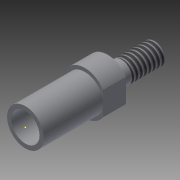
# Autodesk Inventor part: Fuel Adjuster
Saved by Autodesk Inventor 2015 (Build 190159000, 159)
## iProperties
Created: 2016-02-20
Part Number: Fuel Adjuster
Material: Generic
Document SubType Name: Modeling
Designer: Owner
Density: 1 g/cm^3
Appearance: Default
Author: Owner
Autodesk Inventor part; units mm, degrees
ref_plane "XZ Plane" through (0, 0, 0) normal (0, 1, 0) x (-1, 0, 0)
ref_plane "XY Plane" through (0, 0, 0) normal (0, 0, 1) x (1, 0, 0)
sketch "Sketch1" plane through (0, 0, 0) normal (0, 0, 1) x (1, 0, 0)
  circle A0 centre (0, 0) radius 1.9685
  dimension "d0" = 3.937
  constraints: 1 centre point, 1 coincident
  measures "d0" diameter of A0
extrude "Extrusion1" add sketch "Sketch1" along normal blind 8.636
sketch "Sketch2" plane through (0, 0, 8.636) normal (0, 0, 1) x (1, 0, 0)
  circle A0 centre (0, 0) radius 4.0005
  dimension "d3" = 8.001
  constraints: 1 centre point, 1 coincident
  measures "d3" diameter of A0
extrude "Extrusion2" add sketch "Sketch2" along normal blind 4.191
sketch "Sketch3" plane through (0, 0, 12.827) normal (0, 0, 1) x (1, 0, 0)
  circle A0 centre (0, 0) radius 4.0005 projected
  circle A1 centre (0, 0) radius 3.3655
  dimension "d6" = 6.731
  constraints: 1 centre point, 1 coincident
  measures "d6" diameter of A1
extrude "Extrusion3" add sketch "Sketch3" along normal blind 10.922 contours A1
sketch "Sketch4" plane through (0, 0, 23.749) normal (0, 0, 1) x (1, 0, 0)
  circle A0 centre (0, 0) radius 2.6035
  dimension "d9" = 5.207
  constraints: 1 centre point, 1 coincident
  measures "d9" diameter of A0
extrude "Extrusion4" cut sketch "Sketch4" against normal blind 5.08
sketch "Sketch5" plane through (0, 0, 23.749) normal (0, 0, 1) x (1, 0, 0)
  point P0 (0, 0)
sketch "Sketch6" plane through (0, 0, 18.669) normal (0, 0, 1) x (1, 0, 0)
  circle A0 centre (0, 0) radius 1.9685
  dimension "d12" = 3.937
  constraints: 1 centre point, 1 coincident
  measures "d12" diameter of A0
hole "Hole1" at (0, 0, 18.669) direction (0, 0, -1) diameter 3.937 depth 4.953
sketch "Sketch7" plane through (0, 0, 13.716) normal (0, 0, 1) x (1, 0, 0)
  circle A0 centre (0, 0) radius 0.7874
  dimension "d20" = 1.5748
  constraints: 1 centre point, 1 coincident
  measures "d20" diameter of A0
extrude "Extrusion5" cut sketch "Sketch7" against normal through all
sketch "Sketch9" plane through (0, 0, 8.636) normal (0, 0, -1) x (-1, 0, 0)
  circle A0 centre (0, 0) radius 4.0005 projected
  line L0 (3.3655, -2.1627) -> (3.3655, 2.1627)
  line L1 (-3.3655, -2.1627) -> (-3.3655, 2.1627)
  constraints: 4 end point, 3 point on circle, 2 vertical
extrude "Extrusion6" cut sketch "Sketch9" against normal blind 4.953 contours A0 L0
sketch "Sketch10" plane through (0, 0, 8.636) normal (0, 0, -1) x (-1, 0, 0)
  arc A0 (3.3655, 2.1627) -> (3.3655, -2.1627) centre (0, 0) ccw projected
  line L0 (-3.3655, -2.1627) -> (-3.3655, 2.1627)
  constraints: 2 end point, 2 point on circle, 1 vertical
extrude "Extrusion7" cut sketch "Sketch10" against normal blind 4.953
thread "Thread1" size "8-32 UNC" class "2B" standard "ANSI Unified Screw Threads" full length
ref_plane "Work Plane1" through (-1.9685, 0, 0) normal (1, 0, 0) x (0, 1, 0)
sketch "Sketch11" plane through (-1.9685, 0, 0) normal (1, 0, 0) x (0, 1, 0)
  line L0 (0, 0) -> (0, 3.2004)
  dimension "d29" = 3.2004
  constraints: 2 end point, 1 vertical
  measures "d29" distance of L0.start L0.end
hole "Hole2" at (-1.9685, 0, 3.2004) direction (1, 0, 0) diameter 1.651 depth 1.9685 tip angle 118
thread "Thread2" size "8-32 UNC" class "2A" standard "ANSI Unified Screw Threads" length 7.62 offset 2.54
body "Solid1"
